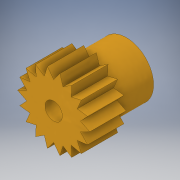
# Autodesk Inventor part: Pignon
Saved by Autodesk Inventor 2019 (Build 230136000, 136)
## iProperties
Created: 2019-07-29
Part Number: Pignon
Material: Laiton, jaune doux, soudé
Document SubType Name: Modeling
Designer: Sébastien DI MERCURIO
Density: 8.5 g/cm^3
Appearance: Soudure - Laiton
Mass: 1.87759 g
Surface Area: 2.06167 cm^2
Volume: 0.220893 cm^3
Author: Sébastien DI MERCURIO
Autodesk Inventor part; units mm, degrees
ref_plane "YZ Plane" through (0, 0, 0) normal (1, 0, 0) x (0, 1, 0)
ref_plane "XZ Plane" through (0, 0, 0) normal (0, 1, 0) x (-1, 0, 0)
ref_plane "XY Plane" through (0, 0, 0) normal (0, 0, 1) x (1, 0, 0)
sketch "Esquisse1" plane through (0, 0, 0) normal (0, 0, 1) x (1, 0, 0)
  circle A0 centre (0, 0) radius 3.75
  dimension "d0" = 7.5
  constraints: 1 centre point, 1 coincident
  measures "d0" diameter of A0
extrude "Extrusion1" add sketch "Esquisse1" along normal blind 5
sketch "Esquisse3" plane through (0, 0, 5) normal (0, 0, 1) x (1, 0, 0)
  circle A0 centre (0, 0) radius 5
  dimension "d12" = 10
  constraints: 1 centre point, 1 coincident
  measures "d12" diameter of A0
extrude "Extrusion2" add sketch "Esquisse3" along normal blind 5
sketch "Esquisse4" plane through (0, 0, 10) normal (0, 0, 1) x (1, 0, 0)
  circle A0 centre (0, 0) radius 3.75
  circle A1 centre (0, 0) radius 5 projected
  circle A2 centre (0, 0) radius 3.75 projected
  line L0 (0, 3.75) -> (-0.9296, 4.9771)
  line L1 (-0.9296, 4.9771) -> (-1, 5.07)
  line L2 (-1, 5.07) -> (1, 5.07)
  line L3 (1, 5.07) -> (0, 3.75)
  dimension "d15" = 7.5
  dimension "d16" = 2
  dimension "d17" = 1.32
  dimension "d18" = 1
  constraints: 8 end point, 1 centre point, 1 coincident, 1 horizontal, 1 point on line, 1 vertical alignment, 1 other
  measures "d15" diameter of A0
  measures "d16" distance of L2.end L1.end
  measures "d17" vertical distance of L0.start L1.end
  measures "d18" horizontal distance of point (0, 0) L1.end
extrude "Extrusion3" cut sketch "Esquisse4" against normal blind 5 contours L0 A1 L3 | L0 L1 L2 L3 A1 picked at (0.3946, 4.554)
pattern_circular "Réseau circulaire1" count 18 over 360 about axis through (0, 0, 5) along (0, 0, 1) of "Extrusion3"
sketch "Esquisse5" plane through (0, 0, 10) normal (0, 0, 1) x (1, 0, 0)
  circle A0 centre (0, 0) radius 1.2
  dimension "d24" = 2.4
  constraints: 1 centre point, 1 coincident
  measures "d24" diameter of A0
extrude "Extrusion4" cut sketch "Esquisse5" against normal through all
sketch "Esquisse6" plane through (0, 0, 0) normal (1, 0, 0) x (0, 1, 0)
  circle A0 centre (0, 3) radius 1.5
  line L0 (-3.75, 0) -> (3.75, 0) projected
  point P0 (0, 0)
  dimension "d27" = 3
  dimension "d28" = 3
  constraints: 1 centre point
  measures "d27" diameter of A0
  measures "d28" distance from line of L0 A0.centre
extrude "Extrusion5" cut sketch "Esquisse6" against normal blind 5
equation "\"d18\" = 0.5 * d16"
